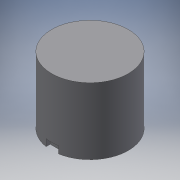
# Autodesk Inventor part: pièce intermédiaire
Saved by Autodesk Inventor 2016 (Build 200138000, 138)
## iProperties
Created: 2016-05-09
Part Number: pièce intermédiaire
Material: Générique
Document SubType Name: Modeling
Designer: Ropert
Density: 1 g/cm^3
Appearance: Par défaut
Author: Ropert
Autodesk Inventor part; units mm, degrees
ref_plane "YZ Plane" through (0, 0, 0) normal (1, 0, 0) x (0, 1, 0)
ref_plane "XZ Plane" through (0, 0, 0) normal (0, 1, 0) x (-1, 0, 0)
ref_plane "XY Plane" through (0, 0, 0) normal (0, 0, 1) x (1, 0, 0)
sketch "Esquisse1" plane through (0, 0, 0) normal (0, 0, 1) x (1, 0, 0)
  circle A0 centre (0, 0) radius 13.5
  circle A1 centre (0, 0) radius 8.25
  dimension "d0" = 27
  dimension "d1" = 16.5
  constraints: 2 centre point, 2 coincident
  measures "d0" diameter of A0
  measures "d1" diameter of A1
extrude "Extrusion1" add sketch "Esquisse1" along normal blind 23.5
sketch "Esquisse2" plane through (0, 0, 23.5) normal (0, 0, 1) x (1, 0, 0)
  circle A0 centre (0, 0) radius 8.25
  constraints: 1 centre point, 1 coincident
extrude "Extrusion2" add sketch "Esquisse2" against normal blind 1.3
sketch "Esquisse3" plane through (0, 0, 0) normal (0, 0, -1) x (-1, 0, 0)
  line L0 (-2.1903, 13.3211) -> (-2.1903, 11.85)
  line L1 (-2.1903, 11.85) -> (0, 11.85)
  line L2 (0, 11.85) -> (2.1903, 11.85)
  line L3 (2.1903, 13.3211) -> (2.1903, 11.85)
  arc A0 (0, 13.5) -> (-2.1903, 13.3211) centre (0, 0) ccw
  arc A1 (2.1903, 13.3211) -> (0, 13.5) centre (0, 0) ccw
  arc A2 (0, -13.5) -> (2.1903, -13.3211) centre (0, 0) ccw
  arc A3 (-2.1903, -13.3211) -> (0, -13.5) centre (0, 0) ccw
  line L4 (-2.1903, -13.3211) -> (-2.1903, -11.85)
  line L5 (0, -11.85) -> (-2.1903, -11.85)
  line L6 (2.1903, -11.85) -> (0, -11.85)
  line L7 (2.1903, -13.3211) -> (2.1903, -11.85)
  point P0 (0, 0)
  point P1 (0, -50)
  point P2 (-13.5, 0)
  constraints: 16 end point, 8 point on circle, 4 centre point, 2 perpendicular
extrude "Extrusion3" cut sketch "Esquisse3" against normal blind 2.5
sketch "Esquisse4" plane through (0, 0, 23.5) normal (0, 0, 1) x (1, 0, 0)
  line L0 (-2.1903, 13.3211) -> (-2.1903, 11.85)
  line L1 (-2.1903, 11.85) -> (0, 11.85)
  line L2 (0, 11.85) -> (2.1903, 11.85)
  line L3 (2.1903, 13.3211) -> (2.1903, 11.85)
  arc A0 (0, 13.5) -> (-2.1903, 13.3211) centre (0, 0) ccw
  arc A1 (2.1903, 13.3211) -> (0, 13.5) centre (0, 0) ccw
  arc A2 (0, -13.5) -> (2.1903, -13.3211) centre (0, 0) ccw
  arc A3 (-2.1903, -13.3211) -> (0, -13.5) centre (0, 0) ccw
  line L4 (-2.1903, -13.3211) -> (-2.1903, -11.85)
  line L5 (0, -11.85) -> (-2.1903, -11.85)
  line L6 (2.1903, -11.85) -> (0, -11.85)
  line L7 (2.1903, -13.3211) -> (2.1903, -11.85)
  point P0 (0, 0)
  point P1 (0, 0)
  constraints: 16 end point, 8 point on circle, 4 centre point, 2 perpendicular
extrude "Extrusion4" cut sketch "Esquisse4" against normal blind 2.5
